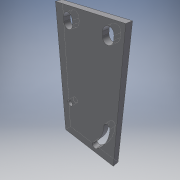
# Autodesk Inventor part: BallBalancing_Hinge
Saved by Autodesk Inventor 2016 (Build 200138000, 138)
## iProperties
Created: 2016-04-08
Part Number: BallBalancing_Hinge
Material: Generic
Document SubType Name: Modeling
Designer: Admin
Density: 1 g/cm^3
Appearance: Default
Author: Admin
Autodesk Inventor part; units mm, degrees
ref_plane "YZ Plane" through (0, 0, 0) normal (1, 0, 0) x (0, 1, 0)
ref_plane "XZ Plane" through (0, 0, 0) normal (0, 1, 0) x (-1, 0, 0)
ref_plane "XY Plane" through (0, 0, 0) normal (0, 0, 1) x (1, 0, 0)
sketch "Sketch1" plane through (0, 0, 0) normal (0, 1, 0) x (-1, 0, 0)
  line L0 (14, 0) -> (-14, 0) projected
  line L1 (0, -48) -> (0, 8) projected
  line L2 (10, -40) -> (-10, -40)
  line L3 (-10, -40) -> (-10, 0)
  line L4 (-10, 0) -> (10, 0)
  line L5 (10, 0) -> (10, -40)
  point P0 (0, 0)
  dimension "d0" = 20
  dimension "d1" = 40
  dimension "d4" = 10
  constraints: 8 end point, 2 parallel, 1 collinear, 1 horizontal, 1 perpendicular
  measures "d0" distance of L2.start L2.end
  measures "d1" distance between parallel lines of L4 L2
  measures "d4" distance between parallel lines of L1 L3
extrude "Extrusion1" add sketch "Sketch1" along normal blind 2
sketch "Sketch2" plane through (0, 2, 0) normal (0, 1, 0) x (1, 0, 0)
  line L0 (10, 40) -> (-10, 40) projected
  line L1 (-10, 40) -> (-10, 0) projected
  line L2 (-10, 0) -> (10, 0) projected
  line L3 (10, 0) -> (10, 40) projected
  line L4 (10, 13.5) -> (-10, 13.5) construction
  line L5 (-10, 13.5) -> (-10, 24.5) construction
  line L6 (-10, 24.5) -> (10, 24.5) construction
  line L7 (10, 24.5) -> (10, 13.5) construction
  line L8 (10, 0) -> (10, 40) projected
  arc A0 (4.5, 8) -> (7.5, 8) centre (6, 8) ccw
  arc A1 (-7.5, 8) -> (-4.5, 8) centre (-6, 8) ccw
  line L9 (0, 49.0401) -> (0, -8.1733) construction
  arc A2 (7.5, 9) -> (4.5, 9) centre (6, 9) ccw
  arc A3 (-4.5, 9) -> (-7.5, 9) centre (-6, 9) ccw
  line L10 (7.5, 8) -> (7.5, 9)
  line L11 (4.5, 8) -> (4.5, 9)
  line L12 (-4.5, 8) -> (-4.5, 9)
  line L13 (-7.5, 8) -> (-7.5, 9)
  circle A4 centre (-7, 27.5) radius 1
  line L14 (-7, 27.5) -> (15.2836, 27.5) construction
  line L15 (-7, 27.5) -> (11.3667, 45.8667) construction
  arc A5 (3.6066, 38.1066) -> (2.1834, 36.6834) centre (2.895, 37.395) ccw
  arc A6 (6, 27.5) -> (8, 27.5) centre (7, 27.5) ccw
  arc A7 (6, 27.5) -> (2.0828, 36.8006) centre (-7, 27.5) ccw
  arc A8 (8, 27.5) -> (3.6066, 38.1066) centre (-7, 27.5) ccw
  point P0 (0, 0)
  dimension "d6" = 11
  dimension "d8" = 3
  dimension "d9" = 3
  dimension "d10" = 8
  dimension "d11" = 8
  dimension "d12" = 6
  dimension "d13" = 6
  dimension "d14" = 3
  dimension "d15" = 3
  dimension "d16" = 4.5
  dimension "d17" = 2
  dimension "d18" = 3
  dimension "d19" = 3
  dimension "d22" = 45
  constraints: 20 end point, 17 point on circle, 9 centre point, 6 point on line, 4 tangent, 3 parallel, 2 coincident, 2 horizontal, 1 collinear, 1 midpoint, 1 perpendicular, 1 vertical
  measures "d6" distance between parallel lines of L4 L6
  measures "d8" diameter of A0
  measures "d9" diameter of A1
  measures "d10" distance from line of L2 A1.centre
  measures "d11" distance from line of L2 A0.centre
  measures "d12" distance from line of L9 A1.centre
  measures "d13" distance from line of L9 A0.centre
  measures "d14" diameter of A2
  measures "d15" diameter of A3
  measures "d16" distance from line of L4 A2.centre
  measures "d17" diameter of A4
  measures "d18" distance from line of L6 L14.start
  measures "d19" distance from line of L1 L14.start
  measures "d22" angle of L14 L15
extrude "Extrusion2" cut sketch "Sketch2" against normal blind 3 contours L11 A2 L10 A0 | L13 A3 L12 A1 | A4 | A8 A6 A7 A5
equation "\"d4\" = 0.5 * d0"
equation "\"d11\" = d10"
equation "\"d13\" = d12"
equation "\"d23\" = d15"
body "Solid1"
